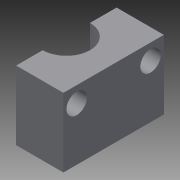
# Autodesk Inventor part: bearing_holder
Saved by Autodesk Inventor 2015 (Build 190159000, 159)
## iProperties
Created: 2017-12-07
Part Number: bearing_holder
Material: Generic
Document SubType Name: Modeling
Designer: Anshul
Density: 1 g/cm^3
Appearance: Default
Author: Anshul
Autodesk Inventor part; units mm, degrees
ref_plane "YZ Plane" through (0, 0, 0) normal (1, 0, 0) x (0, 1, 0)
ref_plane "XZ Plane" through (0, 0, 0) normal (0, 1, 0) x (-1, 0, 0)
ref_plane "XY Plane" through (0, 0, 0) normal (0, 0, 1) x (1, 0, 0)
sketch "Sketch1" plane through (0, 0, 0) normal (0, 1, 0) x (-1, 0, 0)
  arc A0 (0, 9.75) -> (0, -9.75) centre (0, 0) ccw
  arc A1 (0, 6) -> (0, -6) centre (0, 0) ccw
  line L0 (0, 9.75) -> (0, 12.75)
  line L1 (0, -9.75) -> (0, -12.75)
  line L2 (0, -12.75) -> (-12, -12.75)
  line L3 (-12, -12.75) -> (-12, 12.75)
  line L4 (-12, 12.75) -> (0, 12.75)
  line L5 (0, 9.75) -> (0, -9.75)
  dimension "d0" = 19.5
  dimension "d1" = 12
  dimension "d2" = 3
  dimension "d3" = 3
  dimension "d4" = 12
  constraints: 12 end point, 4 point on circle, 4 point on line, 3 perpendicular, 2 centre point, 2 coincident, 1 collinear, 1 vertical
  measures "d0" diameter of A0
  measures "d1" diameter of A1
  measures "d2" distance of L0.start L0.end
  measures "d3" distance of L1.start L1.end
  measures "d4" distance of L1.end L2.end
extrude "Extrusion4" add sketch "Sketch1" along normal blind 11 and the other way blind 6.5 contours L5 A1 A0 | A0 L1 L2 L3 L4 L0
extrude "Extrusion5" cut sketch "Sketch1" along normal blind 3 and the other way blind 3.5 contours L5 A1 A0
sketch "Sketch3" plane through (0, -6.5, 12.75) normal (-1, 0, 0) x (0, 0, 1)
  line L0 (-25.5, 17.5) -> (-18.75, 17.5)
  line L1 (-22.125, 17.5) -> (-22.125, 9.5)
  line L2 (-3, 9.5) -> (-22.5, 9.5) projected
  line L3 (0, 17.5) -> (-6.75, 17.5)
  line L4 (-6.75, 17.5) -> (0, 17.5) projected
  line L5 (-3.375, 17.5) -> (-3.375, 9.5)
  circle A0 centre (-22.125, 13.5) radius 2.6
  circle A1 centre (-3.375, 13.5) radius 2.6
  point P0 (-12.75, 6.5)
  dimension "d23" = 5.2
  dimension "d24" = 5.2
  constraints: 8 end point, 4 midpoint, 2 centre point, 2 perpendicular, 2 point on line, 1 collinear, 1 horizontal
  measures "d23" diameter of A0
  measures "d24" diameter of A1
extrude "Extrusion6" cut sketch "Sketch3" against normal blind 30
body "Solid2"
